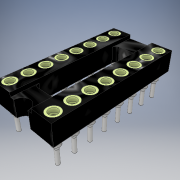
# Autodesk Inventor part: DIL16-Socket
Saved by Autodesk Inventor 2018 (Build 220112000, 112)
## iProperties
Created: 2020-04-18
Part Number: DIL16-Socket
Material: Všeobecné
Document SubType Name: Modeling
Designer: Jozko Mrkvicka
Density: 1 g/cm^3
Appearance: Výchozí
Author: Jozko Mrkvicka
Autodesk Inventor part; units mm, degrees
ref_plane "YZ Plane" through (0, 0, 0) normal (1, 0, 0) x (0, 1, 0)
ref_plane "XZ Plane" through (0, 0, 0) normal (0, 1, 0) x (-1, 0, 0)
ref_plane "XY Plane" through (0, 0, 0) normal (0, 0, 1) x (1, 0, 0)
sketch "Náčrt1" plane through (0, 0, 0) normal (0, 1, 0) x (-1, 0, 0)
  line L0 (10.16, 0) -> (10.16, -20.32)
  line L1 (10.16, -20.32) -> (0, -20.32)
  line L2 (0, -20.32) -> (0, 0)
  line L3 (0, 0) -> (3.175, 0)
  line L4 (3.175, -20.32) -> (0, -20.32)
  line L5 (0, -20.32) -> (0, 0)
  line L6 (10.16, 0) -> (6.985, 0)
  line L7 (6.985, -20.32) -> (10.16, -20.32)
  line L8 (10.16, -20.32) -> (10.16, 0)
  line L9 (3.81, -3.175) -> (6.35, -3.175)
  line L10 (6.985, -20.32) -> (3.175, -20.32)
  line L11 (3.81, -17.145) -> (6.35, -17.145)
  line L12 (6.985, -3.81) -> (6.985, -16.51)
  line L13 (3.175, -3.81) -> (3.175, -16.51)
  arc A0 (3.81, 0) -> (6.35, 0) centre (5.08, 0) ccw
  line L14 (0, 0) -> (3.81, 0)
  line L15 (6.35, 0) -> (10.16, 0)
  line L16 (6.985, 0) -> (6.35, 0)
  line L17 (3.81, 0) -> (3.175, 0)
  arc A1 (6.985, -3.81) -> (6.35, -3.175) centre (6.35, -3.81) ccw
  arc A2 (3.81, -3.175) -> (3.175, -3.81) centre (3.81, -3.81) ccw
  arc A3 (3.175, -16.51) -> (3.81, -17.145) centre (3.81, -16.51) ccw
  arc A4 (6.35, -17.145) -> (6.985, -16.51) centre (6.35, -16.51) ccw
  dimension "d0" = 10.16
  dimension "d1" = 20.32
  dimension "d6" = 2.54
  dimension "d7" = 0.635
  dimension "d111" = 3.175
  dimension "d112" = 3.175
  constraints: 36 end point, 10 point on circle, 9 parallel, 8 horizontal, 8 tangent, 5 centre point, 4 perpendicular, 3 equal radius, 2 point on line
  measures "d0" distance of L0.end L1.end
  measures "d1" distance of L0.start L0.end
  measures "d6" diameter of A0
  measures "d7" radius of A1
  measures "d111" distance between parallel lines of L1 L11
  measures "d112" distance between parallel lines of L3 L9
extrude "Vysunutí8" add sketch "Náčrt1" along normal blind 3.175
sketch "Náčrt8" plane through (0, 3.175, 0) normal (0, 1, 0) x (1, 0, 0)
  line L0 (-3.81, 0) -> (0, 0) projected
  line L1 (-6.985, 21.333) -> (-3.175, 21.333)
  line L2 (-3.175, 21.333) -> (-3.175, 0)
  line L3 (-3.175, 0) -> (-6.985, 0)
  line L4 (-6.985, 0) -> (-6.985, 21.333)
  constraints: 8 end point, 2 parallel, 1 horizontal, 1 perpendicular, 1 point on line
extrude "Vysunutí9" cut sketch "Náčrt8" against normal blind 0.635
sketch "Náčrt9" plane through (0, 3.175, 0) normal (0, 1, 0) x (1, 0, 0)
  circle A0 centre (-1.27, 19.05) radius 0.635
  circle A1 centre (-1.27, 16.51) radius 0.635
  circle A2 centre (-1.27, 13.97) radius 0.635
  circle A3 centre (-1.27, 11.43) radius 0.635
  circle A4 centre (-1.27, 8.89) radius 0.635
  circle A5 centre (-1.27, 6.35) radius 0.635
  circle A6 centre (-1.27, 3.81) radius 0.635
  circle A7 centre (-1.27, 1.27) radius 0.635
  circle A8 centre (-8.89, 19.05) radius 0.635
  circle A9 centre (-8.89, 16.51) radius 0.635
  circle A10 centre (-8.89, 13.97) radius 0.635
  circle A11 centre (-8.89, 1.27) radius 0.635
  circle A12 centre (-8.89, 3.81) radius 0.635
  circle A13 centre (-8.89, 6.35) radius 0.635
  circle A14 centre (-8.89, 8.89) radius 0.635
  circle A15 centre (-8.89, 11.43) radius 0.635
  point P0 (0, 0)
  point P1 (-8.89, 19.05)
  point P2 (-8.89, 16.51)
  point P3 (-8.89, 11.43)
  point P4 (-8.89, 8.89)
  point P5 (-8.89, 6.35)
  point P6 (-8.89, 3.81)
  point P7 (-8.89, 1.27)
  point P8 (-1.27, 1.27)
  point P9 (-1.27, 3.81)
  point P10 (-1.27, 6.35)
  point P11 (-1.27, 8.89)
  point P12 (-1.27, 11.43)
  point P13 (-1.27, 1.27)
  constraints: 16 centre point
extrude "Vysunutí10" cut sketch "Náčrt9" against normal blind 0.635
sketch "Náčrt10" plane through (-8.89, 2.54, -1.27) normal (0, 1, 0) x (1, 0, 0)
  circle A0 centre (7.62, 17.78) radius 0.3175
  circle A1 centre (7.62, 17.78) radius 0.3175
  circle A2 centre (7.62, 15.24) radius 0.3175
  circle A3 centre (7.62, 15.24) radius 0.3175
  circle A4 centre (7.62, 12.7) radius 0.3175
  circle A5 centre (7.62, 12.7) radius 0.3175
  circle A6 centre (7.62, 10.16) radius 0.3175
  circle A7 centre (7.62, 10.16) radius 0.3175
  circle A8 centre (7.62, 7.62) radius 0.3175
  circle A9 centre (7.62, 5.08) radius 0.3175
  circle A10 centre (7.62, 5.08) radius 0.3175
  circle A11 centre (7.62, 2.54) radius 0.3175
  circle A12 centre (7.62, 0) radius 0.3175
  circle A13 centre (7.62, 0) radius 0.3175
  circle A14 centre (0, 0) radius 0.3175
  circle A15 centre (0, 0) radius 0.3175
  circle A16 centre (0, 2.54) radius 0.3175
  circle A17 centre (0, 5.08) radius 0.3175
  circle A18 centre (0, 7.62) radius 0.3175
  circle A19 centre (0, 7.62) radius 0.3175
  circle A20 centre (0, 10.16) radius 0.3175
  circle A21 centre (0, 10.16) radius 0.3175
  circle A22 centre (0, 12.7) radius 0.3175
  circle A23 centre (0, 15.24) radius 0.3175
  circle A24 centre (0, 15.24) radius 0.3175
  circle A25 centre (0, 17.78) radius 0.3175
  circle A26 centre (0, 17.78) radius 0.3175
  point P0 (8.89, -1.27)
  constraints: 27 centre point, 15 coincident
extrude "Vysunutí11" cut sketch "Náčrt10" against normal blind 1.27
sketch "Náčrt11" plane through (0, 3.175, 0) normal (0, 1, 0) x (1, 0, 0)
  circle A0 centre (-8.89, 1.27) radius 0.9525
  circle A1 centre (-8.89, 8.89) radius 0.9525
  circle A2 centre (-8.89, 3.81) radius 0.9525
  circle A3 centre (-8.89, 6.35) radius 0.9525
  circle A4 centre (-8.89, 11.43) radius 0.9525
  circle A5 centre (-8.89, 13.97) radius 0.9525
  circle A6 centre (-8.89, 16.51) radius 0.9525
  circle A7 centre (-8.89, 19.05) radius 0.9525
  circle A8 centre (-1.27, 1.27) radius 0.9525
  circle A9 centre (-1.27, 3.81) radius 0.9525
  circle A10 centre (-1.27, 6.35) radius 0.9525
  circle A11 centre (-1.27, 8.89) radius 0.9525
  circle A12 centre (-1.27, 11.43) radius 0.9525
  circle A13 centre (-1.27, 13.97) radius 0.9525
  circle A14 centre (-1.27, 16.51) radius 0.9525
  circle A15 centre (-1.27, 19.05) radius 0.9525
  constraints: 16 centre point
extrude "Vysunutí12" cut sketch "Náčrt11" against normal blind 0.0254
sketch "Náčrt12" plane through (0, 0, 0) normal (0, -1, 0) x (1, 0, 0)
  circle A0 centre (-8.89, -6.35) radius 0.635 projected
  circle A1 centre (-8.89, -1.27) radius 0.635 projected
  circle A2 centre (-8.89, -3.81) radius 0.635 projected
  circle A3 centre (-8.89, -8.89) radius 0.635 projected
  circle A4 centre (-8.89, -11.43) radius 0.635 projected
  circle A5 centre (-8.89, -13.97) radius 0.635 projected
  circle A6 centre (-8.89, -16.51) radius 0.635 projected
  circle A7 centre (-8.89, -19.05) radius 0.635 projected
  circle A8 centre (-1.27, -1.27) radius 0.635 projected
  circle A9 centre (-1.27, -3.81) radius 0.635 projected
  circle A10 centre (-1.27, -6.35) radius 0.635 projected
  circle A11 centre (-1.27, -8.89) radius 0.635 projected
  circle A12 centre (-1.27, -11.43) radius 0.635 projected
  circle A13 centre (-1.27, -13.97) radius 0.635 projected
  circle A14 centre (-1.27, -16.51) radius 0.635 projected
  circle A15 centre (-1.27, -19.05) radius 0.635 projected
  point P0 (0, 0)
extrude "Vysunutí13" add sketch "Náčrt12" along normal blind 1.905
chamfer "Zkosení29" distance 0.3175 distance2 0.635 1 edges at (-1.905, -1.905, -1.27) measured on face at (-1.0935, -1.905, -1.2787)
chamfer "Zkosení30" distance 0.3175 distance2 0.635 1 edges at (-1.905, -1.905, -3.81) measured on face at (-1.0282, -1.905, -4.0079)
chamfer "Zkosení31" distance 0.3175 distance2 0.635 1 edges at (-1.905, -1.905, -6.35) measured on face at (-1.0645, -1.905, -6.4007)
chamfer "Zkosení32" distance 0.3175 distance2 0.635 1 edges at (-1.905, -1.905, -8.89) measured on face at (-1.4636, -1.905, -8.9377)
chamfer "Zkosení33" distance 0.3175 distance2 0.635 1 edges at (-1.905, -1.905, -11.43) measured on face at (-1.4636, -1.905, -11.4777)
chamfer "Zkosení34" distance 0.3175 distance2 0.635 1 edges at (-1.905, -1.905, -13.97) measured on face at (-1.4636, -1.905, -14.0177)
chamfer "Zkosení35" distance 0.3175 distance2 0.635 1 edges at (-1.905, -1.905, -16.51) measured on face at (-1.0826, -1.905, -16.5129)
chamfer "Zkosení36" distance 0.3175 distance2 0.635 1 edges at (-1.905, -1.905, -19.05) measured on face at (-1.0826, -1.905, -19.0529)
chamfer "Zkosení37" distance 0.3175 distance2 0.635 1 edges at (-9.525, -1.905, -19.05) measured on face at (-8.7026, -1.905, -18.9516)
chamfer "Zkosení38" distance 0.3175 distance2 0.635 1 edges at (-9.525, -1.905, -16.51) measured on face at (-8.7026, -1.905, -16.4116)
chamfer "Zkosení39" distance 0.3175 distance2 0.635 1 edges at (-9.525, -1.905, -13.97) measured on face at (-8.6783, -1.905, -14.1667)
chamfer "Zkosení40" distance 0.3175 distance2 0.635 1 edges at (-9.525, -1.905, -11.43) measured on face at (-8.6783, -1.905, -11.6267)
chamfer "Zkosení41" distance 0.3175 distance2 0.635 1 edges at (-9.525, -1.905, -8.89) measured on face at (-8.6783, -1.905, -9.0867)
chamfer "Zkosení42" distance 0.3175 distance2 0.635 1 edges at (-9.525, -1.905, -6.35) measured on face at (-8.6964, -1.905, -6.499)
chamfer "Zkosení43" distance 0.3175 distance2 0.635 1 edges at (-9.525, -1.905, -3.81) measured on face at (-8.6964, -1.905, -3.959)
chamfer "Zkosení44" distance 0.3175 distance2 0.635 1 edges at (-9.525, -1.905, -1.27) measured on face at (-8.6964, -1.905, -1.419)
sketch "Náčrt13" plane through (-8.89, -1.905, -19.05) normal (0, -1, 0) x (1, 0, 0)
  circle A0 centre (7.62, 0) radius 0.3175 projected
  circle A1 centre (7.62, 2.54) radius 0.3175 projected
  circle A2 centre (7.62, 5.08) radius 0.3175 projected
  circle A3 centre (7.62, 7.62) radius 0.3175 projected
  circle A4 centre (7.62, 10.16) radius 0.3175 projected
  circle A5 centre (7.62, 12.7) radius 0.3175 projected
  circle A6 centre (7.62, 15.24) radius 0.3175 projected
  circle A7 centre (7.62, 17.78) radius 0.3175 projected
  circle A8 centre (0, 0) radius 0.3175 projected
  circle A9 centre (0, 2.54) radius 0.3175 projected
  circle A10 centre (0, 5.08) radius 0.3175 projected
  circle A11 centre (0, 7.62) radius 0.3175 projected
  circle A12 centre (0, 10.16) radius 0.3175 projected
  circle A13 centre (0, 12.7) radius 0.3175 projected
  circle A14 centre (0, 15.24) radius 0.3175 projected
  circle A15 centre (0, 17.78) radius 0.3175 projected
  point P0 (8.89, 19.05)
extrude "Vysunutí14" add sketch "Náčrt13" along normal blind 2.54
fillet "Zaoblení2" radius 0.127 16 edges at (-9.2075, -4.445, -19.05) (-9.2075, -4.445, -16.51) (-9.2075, -4.445, -13.97) (-9.2075, -4.445, -11.43) (-9.2075, -4.445, -8.89) (-9.2075, -4.445, -6.35) (-9.2075, -4.445, -3.81) (-9.2075, -4.445, -1.27) (-1.5875, -4.445, -1.27) (-1.5875, -4.445, -3.81) (-1.5875, -4.445, -6.35) (-1.5875, -4.445, -8.89) (-1.5875, -4.445, -11.43) (-1.5875, -4.445, -13.97) (-1.5875, -4.445, -16.51) (-1.5875, -4.445, -19.05)
